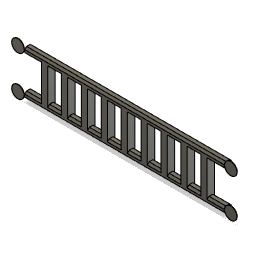
Leiter_TipToi_Feuerwehr (Autodesk Fusion 360 design; units mm, degrees)
Autodesk Fusion 360 part; units mm, degrees
note: some values were not read from the file. Set by a fixed rule: which sketch regions a step uses.
sketch "Skizze1" plane through (0, 0, 0) normal (0, 0, 1) x (1, 0, 0)
  line L0 (2.5, 13) -> (-2.5, 13)
  line L1 (-2.5, 13) -> (-2.5, -13)
  line L2 (-2.5, -13) -> (2.5, -13)
  line L3 (2.5, -13) -> (2.5, 13)
  line L4 (2.5, 13) -> (-2.5, -13) construction
  line L5 (-2.5, 13) -> (2.5, -13) construction
  line L6 (80, 13) -> (-80, 13)
  line L7 (-80, 13) -> (-80, 18)
  line L8 (-80, 18) -> (80, 18)
  line L9 (80, 18) -> (80, 13)
  line L10 (80, 13) -> (-80, 18) construction
  line L11 (-80, 13) -> (80, 18) construction
  line L12 (80, -18) -> (-80, -18)
  line L13 (-80, -18) -> (-80, -13)
  line L14 (-80, -13) -> (80, -13)
  line L15 (80, -13) -> (80, -18)
  line L16 (80, -18) -> (-80, -13) construction
  line L17 (-80, -18) -> (80, -13) construction
  line L18 (-61.5, 13) -> (-66.5, 13)
  line L19 (-61.5, -13) -> (-61.5, 13)
  line L20 (-61.5, 13) -> (-66.5, -13) construction
  line L21 (-66.5, 13) -> (-61.5, -13) construction
  line L22 (-66.5, -13) -> (-61.5, -13)
  line L23 (-66.5, 13) -> (-66.5, -13)
  line L24 (-45.5, 13) -> (-50.5, 13)
  line L25 (-45.5, -13) -> (-45.5, 13)
  line L26 (-45.5, 13) -> (-50.5, -13) construction
  line L27 (-50.5, 13) -> (-45.5, -13) construction
  line L28 (-50.5, -13) -> (-45.5, -13)
  line L29 (-50.5, 13) -> (-50.5, -13)
  line L30 (-29.5, 13) -> (-34.5, 13)
  line L31 (-29.5, -13) -> (-29.5, 13)
  line L32 (-29.5, 13) -> (-34.5, -13) construction
  line L33 (-34.5, 13) -> (-29.5, -13) construction
  line L34 (-34.5, -13) -> (-29.5, -13)
  line L35 (-34.5, 13) -> (-34.5, -13)
  line L36 (-13.5, 13) -> (-18.5, 13)
  line L37 (-13.5, -13) -> (-13.5, 13)
  line L38 (-13.5, 13) -> (-18.5, -13) construction
  line L39 (-18.5, 13) -> (-13.5, -13) construction
  line L40 (-18.5, -13) -> (-13.5, -13)
  line L41 (-18.5, 13) -> (-18.5, -13)
  line L42 (18.5, 13) -> (13.5, 13)
  line L43 (18.5, -13) -> (18.5, 13)
  line L44 (18.5, 13) -> (13.5, -13) construction
  line L45 (13.5, 13) -> (18.5, -13) construction
  line L46 (13.5, -13) -> (18.5, -13)
  line L47 (13.5, 13) -> (13.5, -13)
  line L48 (34.5, 13) -> (29.5, 13)
  line L49 (34.5, -13) -> (34.5, 13)
  line L50 (34.5, 13) -> (29.5, -13) construction
  line L51 (29.5, 13) -> (34.5, -13) construction
  line L52 (29.5, -13) -> (34.5, -13)
  line L53 (29.5, 13) -> (29.5, -13)
  line L54 (50.5, 13) -> (45.5, 13)
  line L55 (50.5, -13) -> (50.5, 13)
  line L56 (50.5, 13) -> (45.5, -13) construction
  line L57 (45.5, 13) -> (50.5, -13) construction
  line L58 (45.5, -13) -> (50.5, -13)
  line L59 (45.5, 13) -> (45.5, -13)
  line L60 (66.5, 13) -> (61.5, 13)
  line L61 (66.5, -13) -> (66.5, 13)
  line L62 (66.5, 13) -> (61.5, -13) construction
  line L63 (61.5, 13) -> (66.5, -13) construction
  line L64 (61.5, -13) -> (66.5, -13)
  line L65 (61.5, 13) -> (61.5, -13)
  point P0 (0, 15.5)
  point P1 (0, -15.5)
  point P2 (-64, 0)
  point P3 (-64, 15.5)
  point P4 (-64, 0)
  point P5 (-64, -15.5)
  point P6 (-48, 0)
  point P7 (-48, 15.5)
  point P8 (-48, 0)
  point P9 (-48, -15.5)
  point P10 (-32, 0)
  point P11 (-32, 15.5)
  point P12 (-32, 0)
  point P13 (-32, -15.5)
  point P14 (-16, 0)
  point P15 (-16, 15.5)
  point P16 (-16, 0)
  point P17 (-16, -15.5)
  point P18 (16, 0)
  point P19 (16, 15.5)
  point P20 (16, 0)
  point P21 (16, -15.5)
  point P22 (32, 0)
  point P23 (32, 15.5)
  point P24 (32, 0)
  point P25 (32, -15.5)
  point P26 (48, 0)
  point P27 (48, 15.5)
  point P28 (48, 0)
  point P29 (48, -15.5)
  point P30 (64, 0)
  point P31 (64, 15.5)
  point P32 (64, 0)
  point P33 (64, -15.5)
  dimension "d1" = 5
  dimension "d2" = 26
  dimension "d3" = 160
  dimension "d6" = 16
  dimension "d7" = 0
  constraint horizontal L0
  constraint perpendicular L0 L1
  constraint parallel L0 L2
  constraint parallel L1 L3
  constraint coincident L4 origin
  constraint coincident L5 origin
  constraint horizontal L6
  constraint perpendicular L6 L7
  constraint parallel L6 L8
  constraint parallel L7 L9
  constraint coincident L10 P0
  constraint coincident L11 P0
  constraint horizontal L12
  constraint perpendicular L12 L13
  constraint parallel L12 L14
  constraint parallel L13 L15
  constraint coincident L16 P1
  constraint coincident L17 P1
  constraint equal L9 L15
  constraint equal L0 L9
  constraint collinear L7 L13
  constraint collinear L9 L15
  constraint collinear L0 L6
  constraint collinear L2 L14
  constraint vertical origin P0
  measures "d1" distance of L1.end L2.end
  measures "d2" distance of L0.end L1.end
  measures "d3" distance of L7.end L8.end
extrude "Extrusion1" add sketch "Skizze1" along normal blind 6 contours L0 L1 L2 L3 L6 L14 | L0 L6 L7 L8 L9 L18 L24 L30 L36 L42 L48 L54 L60 | L2 L12 L13 L14 L15 L22 L28 L34 L40 L46 L52 L58 L64 | L6 L14 L42 L43 L46 L47 | L6 L14 L36 L37 L40 L41 | L6 L14 L48 L49 L52 L53 | L6 L14 L30 L31 L34 L35 | L6 L14 L54 L55 L58 L59 | L6 L14 L24 L25 L28 L29 | L6 L14 L60 L61 L64 L65 | L6 L14 L18 L19 L22 L23
chamfer "Fase1" distance 1.5 angle 45 44 edges at (0, 18, 0) (0, 18, 6) (0, -18, 6) (0, -18, 0) (-73.25, 13, 6) (-56, 13, 6) (-40, 13, 6) (-40, 13, 0) (-56, 13, 0) (-73.25, 13, 0) (-24, 13, 6) (-24, 13, 0) (-8, 13, 6) (-8, 13, 0) (8, 13, 6) (8, 13, 0) (24, 13, 6) (24, 13, 0) (40, 13, 6) (40, 13, 0) (56, 13, 6) (56, 13, 0) (73.25, 13, 6) (73.25, 13, 0) (73.25, -13, 6) (56, -13, 6) (40, -13, 6) (24, -13, 6) (8, -13, 6) (-8, -13, 6) (-24, -13, 6) (-40, -13, 6) (-56, -13, 6) (-73.25, -13, 6) (-73.25, -13, 0) (-56, -13, 0) (-40, -13, 0) (-24, -13, 0) (-8, -13, 0) (8, -13, 0) (24, -13, 0) (40, -13, 0) (56, -13, 0) (73.25, -13, 0)
sketch "Skizze2" plane through (0, 0, 6) normal (0, 0, 1) x (1, 0, 0)
  line L0 (-66.5, -14.5) -> (-80, -14.5)
  line L1 (-80, -14.5) -> (-80, -16.5)
  line L2 (-80, -16.5) -> (80, -16.5)
  line L3 (80, -16.5) -> (80, -14.5)
  line L4 (80, -14.5) -> (66.5, -14.5)
  line L5 (66.5, -14.5) -> (66.5, 14.5)
  line L6 (66.5, 14.5) -> (80, 14.5)
  line L7 (80, 14.5) -> (80, 16.5)
  line L8 (80, 16.5) -> (-80, 16.5)
  line L9 (-80, 16.5) -> (-80, 14.5)
  line L10 (-80, 14.5) -> (-66.5, 14.5)
  line L11 (-66.5, 14.5) -> (-66.5, -14.5)
  line L12 (-61.5, -14.5) -> (-61.5, 14.5)
  line L13 (-61.5, 14.5) -> (-50.5, 14.5)
  line L14 (-50.5, 14.5) -> (-50.5, -14.5)
  line L15 (-50.5, -14.5) -> (-61.5, -14.5)
  line L16 (-45.5, -14.5) -> (-45.5, 14.5)
  line L17 (-45.5, 14.5) -> (-34.5, 14.5)
  line L18 (-34.5, 14.5) -> (-34.5, -14.5)
  line L19 (-34.5, -14.5) -> (-45.5, -14.5)
  line L20 (-29.5, -14.5) -> (-29.5, 14.5)
  line L21 (-29.5, 14.5) -> (-18.5, 14.5)
  line L22 (-18.5, 14.5) -> (-18.5, -14.5)
  line L23 (-18.5, -14.5) -> (-29.5, -14.5)
  line L24 (-13.5, -14.5) -> (-13.5, 14.5)
  line L25 (-13.5, 14.5) -> (-2.5, 14.5)
  line L26 (-2.5, 14.5) -> (-2.5, -14.5)
  line L27 (-2.5, -14.5) -> (-13.5, -14.5)
  line L28 (2.5, -14.5) -> (2.5, 14.5)
  line L29 (2.5, 14.5) -> (13.5, 14.5)
  line L30 (13.5, 14.5) -> (13.5, -14.5)
  line L31 (13.5, -14.5) -> (2.5, -14.5)
  line L32 (18.5, -14.5) -> (18.5, 14.5)
  line L33 (18.5, 14.5) -> (29.5, 14.5)
  line L34 (29.5, 14.5) -> (29.5, -14.5)
  line L35 (29.5, -14.5) -> (18.5, -14.5)
  line L36 (34.5, -14.5) -> (34.5, 14.5)
  line L37 (34.5, 14.5) -> (45.5, 14.5)
  line L38 (45.5, 14.5) -> (45.5, -14.5)
  line L39 (45.5, -14.5) -> (34.5, -14.5)
  line L40 (50.5, -14.5) -> (50.5, 14.5)
  line L41 (50.5, 14.5) -> (61.5, 14.5)
  line L42 (61.5, 14.5) -> (61.5, -14.5)
  line L43 (61.5, -14.5) -> (50.5, -14.5)
  circle A0 centre (-85.5, 16.5) radius 5
  circle A1 centre (-85.5, -15.5) radius 5
  circle A2 centre (85.5, 16.5) radius 5
  circle A3 centre (85.5, -14.5) radius 5
  line L44 (-80, 16.5) -> (-85.5, 16.5)
  line L45 (-85.5, 16.5) -> (-85.5, 15.5)
  line L46 (-85.5, 15.5) -> (-80, 15.5)
  line L47 (-80, 15.5) -> (-80, 16.5)
  line L48 (-80, -14.5) -> (-85.5, -14.5)
  line L49 (-85.5, -14.5) -> (-85.5, -15.5)
  line L50 (-85.5, -15.5) -> (-80, -15.5)
  line L51 (-80, -15.5) -> (-80, -14.5)
  line L52 (80, 16.5) -> (85.5, 16.5)
  line L53 (85.5, 16.5) -> (85.5, 15.5)
  line L54 (85.5, 15.5) -> (80, 15.5)
  line L55 (80, 15.5) -> (80, 16.5)
  line L56 (80, -14.5) -> (85.5, -14.5)
  line L57 (85.5, -14.5) -> (85.5, -15.5)
  line L58 (85.5, -15.5) -> (80, -15.5)
  line L59 (80, -15.5) -> (80, -14.5)
  dimension "d11" = 10
  dimension "d12" = 1
  dimension "d13" = 5.5
  constraint horizontal L44
  constraint vertical L45
  constraint horizontal L46
  constraint vertical L47
  constraint coincident L8.end L9.start
  constraint horizontal L48
  constraint vertical L49
  constraint horizontal L50
  constraint vertical L51
  constraint coincident A1.centre L49.end
  constraint coincident L0.end L1.start
  constraint horizontal L52
  constraint vertical L53
  constraint horizontal L54
  constraint vertical L55
  constraint coincident L7.end L8.start
  constraint horizontal L56
  constraint vertical L57
  constraint horizontal L58
  constraint vertical L59
  constraint coincident L3.end L4.start
  constraint coincident A3.centre L56.end
  constraint vertical A2.centre A3.centre
  constraint vertical A0.centre A1.centre
  constraint equal A0 A2
  constraint equal A2 A3
  constraint equal A1 A3
  constraint equal L45 L49
  constraint equal L49 L57
  constraint equal L53 L57
  constraint coincident A2.centre L52.end
  constraint equal L44 L52
  constraint coincident A0.centre L44.end
  measures "d11" diameter of A0
  measures "d12" distance of L44 L46
  measures "d13" distance of L7.end A2.centre
extrude "Extrusion2" add sketch "Skizze2" against normal blind 0.3 contours L1 A1 L48 L50 L51 | A1 L48 L49 L50 | A1 L48 L49 L50 | L9 A0 L44 L46 L47 | A0 L44 L45 L46 | A0 L44 L45 L46 | L3 A3 L56 L58 L59 | L7 A2 L52 L54 L55 | A3 L56 L57 L58 | A3 L56 L57 L58 | A2 L52 L53 L54 | A2 L52 L53 L54
